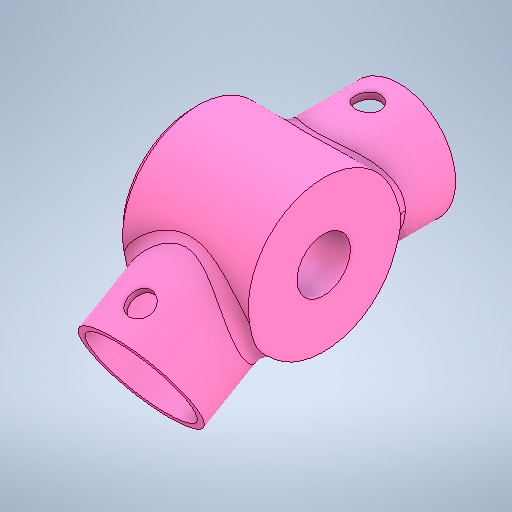
# Autodesk Inventor part: bielle rocker2
Saved by Autodesk Inventor 2026.2 (Build 302298010, 298A)
## iProperties
Created: 2026-03-19
Part Number: bielle rocker2
Material: Générique
Document SubType Name: Modeling
Designer: Genon
Density: 1 g/cm^3
Appearance: Rose
Author: Genon
Autodesk Inventor part; units mm, degrees
ref_plane "YZ Plane" through (0, 0, 0) normal (1, 0, 0) x (0, 1, 0)
sketch "Esquisse1" plane through (0, 0, 0) normal (1, 0, 0) x (0, 1, 0)
  circle A0 centre (0, 0) radius 12
  circle A1 centre (0, 0) radius 4.25
  dimension "d0" = 24
  dimension "d1" = 8.5
  constraints: 2 centre point, 2 coincident
  measures "d0" diameter of A0
  measures "d1" diameter of A1
extrude "Extrusion1" add sketch "Esquisse1" against normal blind 20
sketch "Esquisse2" plane through (-20, 0, 0) normal (-1, 0, 0) x (0, 0, 1)
  circle A0 centre (0, 0) radius 4.25 projected
  circle A1 centre (0, 0) radius 10.95
  dimension "d4" = 21.9
  constraints: 1 centre point, 1 coincident
  measures "d4" diameter of A1
extrude "Extrusion2" add sketch "Esquisse2" along normal blind 1
ref_plane "Plan de construction5" through (0, 0, -12) normal (0, 0, 1) x (1, 0, 0)
sketch "Esquisse14" plane through (0, 0, -12) normal (0, 0, 1) x (1, 0, 0)
  line L0 (0, 0) -> (-10, 0)
  circle A0 centre (-10, 0) radius 8
  circle A1 centre (-10, 0) radius 9
  dimension "d46" = 10
  dimension "d47" = 16
  dimension "d48" = 18
  constraints: 2 centre point, 2 coincident, 2 end point, 1 horizontal
  measures "d46" distance of L0.start L0.end
  measures "d47" diameter of A0
  measures "d48" diameter of A1
extrude "Extrusion10" add sketch "Esquisse14" against normal blind 10
sketch "Esquisse15" plane through (0, 0, -12) normal (0, 0, 1) x (1, 0, 0)
  circle A0 centre (-10, 0) radius 8 projected
  circle A1 centre (-10, 0) radius 9 projected
  point P0 (0, 0)
extrude "Extrusion11" add sketch "Esquisse15" along normal blind 5 contours A0 | A1
ref_plane "Plan de construction7" through (0, -6, 10.392305) normal (0, -0.5, 0.8660254) x (1, 0, 0)
ref_plane "Plan de construction6" through (0, 0, 0) normal (0, -0.5, 0.8660254) x (1, 0, 0)
sketch "Esquisse16" plane through (0, -6, 10.392305) normal (0, -0.5, 0.8660254) x (1, 0, 0)
  line L0 (0, 0) -> (-10, 0)
  ellipse E0 centre (-10, -6) end of major axis (-18, -6) minor radius 6.928203
  line L1 (0, 0) -> (10, 0) construction
  circle A0 centre (-10, 0) radius 8
  circle A1 centre (-10, 0) radius 9
  dimension "d55" = 10
  dimension "d56" = 180
  dimension "d57" = 16
  dimension "d58" = 18
  constraints: 4 end point, 2 centre point, 2 coincident, 2 horizontal, 1 collinear, 1 other
  measures "d55" distance of L0.start L0.end
  measures "d56" angle of L0 L1
  measures "d57" diameter of A0
  measures "d58" diameter of A1
extrude "Extrusion12" add sketch "Esquisse16" along normal blind 10 contours A1 E0 A0 L0 | L0 A0 E0 A1 | E0 A0 A1
sketch "Esquisse17" plane through (0, -6, 10.392305) normal (0, -0.5, 0.8660254) x (1, 0, 0)
  circle A0 centre (-10, 0) radius 8 projected
  circle A1 centre (-10, 0) radius 9 projected
  point P0 (0, 0)
  constraints: 1 horizontal alignment
extrude "Extrusion13" add sketch "Esquisse17" against normal blind 5 contours A0 | A1
ref_plane "Plan de construction8" through (0, 0, 0) normal (0, -0.8660254, -0.5) x (1, 0, 0)
sketch "Esquisse18" plane through (0, 0, 0) normal (0, -0.8660254, -0.5) x (1, 0, 0)
  line L0 (-1, 22) -> (-19, 22) projected
  line L1 (-19, 22) -> (-10, 22)
  line L2 (-10, 22) -> (-10, 17)
  point P0 (0, 0)
  dimension "d64" = 9
  dimension "d65" = 5
  constraints: 4 end point, 1 coincident, 1 midpoint, 1 perpendicular
  measures "d64" distance of L0.end L1.end
  measures "d65" distance of L1.end L2.end
hole "Perçage2" at (-10, -8.5, 14.722432) direction (0, 0.8660254, 0.5) diameter 4 end through all both
sketch "Esquisse19" plane through (0, 0, 0) normal (0, 1, 0) x (-1, 0, 0)
  line L0 (1, -12) -> (1, -22) projected
  line L1 (1, -22) -> (10, -22)
  line L2 (18, -22) -> (2, -22) projected
  line L3 (1, -22) -> (10, -22) construction
  line L4 (10, -22) -> (10, -17)
  point P0 (0, 0)
  dimension "d73" = 9
  dimension "d74" = 0
  dimension "d75" = 5
  constraints: 6 end point, 2 collinear, 1 coincident, 1 horizontal, 1 perpendicular, 1 point on line
  measures "d73" distance of L1.start L1.end
  measures "d74" distance between parallel lines of L1 L3
  measures "d75" distance of L1.end L4.end
hole "Perçage3" at (-10, 0, -17) direction (0, -1, 0) diameter 4 end through all both
fillet "Congé2" radius 2 4 edges at (-10.0136, -11.7629, 2.3739) (-10.0134, 3.8256, 11.3739) (-10.0136, -9, -7.9373) (-10.0134, 9, -7.9373)
